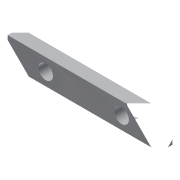
# Autodesk Inventor part: Bearing Retention Plate
Saved by Autodesk Inventor 2014 SP1 (Build 180222100, 222)
## iProperties
Created: 2014-05-15
Part Number: Bearing Retention Plate
Material: Aluminum 6061
Document SubType Name: Modeling
Designer: Rauhul Varma
Density: 2.71 g/cm^3
Appearance: Aluminum - Flat
Mass: 1.90086 g
Surface Area: 7.97065 cm^2
Volume: 0.701424 cm^3
Author: Rauhul Varma
Autodesk Inventor part; units mm, degrees
ref_plane "YZ Plane" through (0, 0, 0) normal (1, 0, 0) x (0, 1, 0)
ref_plane "XZ Plane" through (0, 0, 0) normal (0, 1, 0) x (-1, 0, 0)
ref_plane "XY Plane" through (0, 0, 0) normal (0, 0, 1) x (1, 0, 0)
sketch "Sketch1" plane through (0, 0, 0) normal (0, 0, 1) x (1, 0, 0)
  line L0 (0, 0) -> (38.1, 0)
  line L1 (38.1, 0) -> (38.1, 6.35)
  line L2 (38.1, 6.35) -> (0, 6.35)
  line L3 (0, 6.35) -> (0, 0)
  line L4 (0, 3.175) -> (38.1, 3.175)
  point P0 (9.525, 3.175)
  point P1 (28.575, 3.175)
  dimension "d0" = 38.1
  dimension "d1" = 19.05
  dimension "d2" = 9.525
  dimension "d3" = 9.525
  dimension "d13" = 6.35
  constraints: 10 end point, 2 midpoint, 2 parallel, 2 point on line, 1 horizontal, 1 perpendicular
  measures "d0" distance of L2.end L1.end
  measures "d1" distance of point (28.575, 3.175) point (9.525, 3.175)
  measures "d2" distance from line of L3 point (9.525, 3.175)
  measures "d3" distance from line of L1 point (28.575, 3.175)
  measures "d13" distance between parallel lines of L0 L2
extrude "Extrusion1" add sketch "Sketch1" against normal blind 3.175
hole "Hole1" at (9.525, 3.175, 0) at (28.575, 3.175, 0) direction (0, 0, -1) diameter 3.6576 end through all clearance for "Flat Head Machine Screw (82)" size "#6" standard "Ansi Unified Screw Threads"
equation "\"d1\" = 0.5 * d0"
equation "\"d2\" = d3"
body "Solid1"
